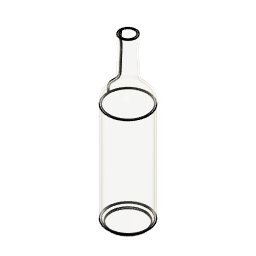
Glass_bottle_ (Autodesk Fusion 360 design; units mm, degrees)
Autodesk Fusion 360 part; units mm, degrees
sketch "Sketch1" plane through (0, 0, 0) normal (0, 1, 0) x (1, 0, 0)
  line L0 (0, 0) -> (0, -240)
  line L1 (0, 0) -> (-29.692, 0)
  line L2 (-29.692, 0) -> (-29.692, -150)
  spline S0 degree 5 poles (-29.692, -150) (-29.8152, -150.759) (-30.0072, -152.2507) (-30.1322, -154.409) (-29.9719, -157.1282) (-29.2328, -160.2645) (-27.979, -163.1461) (-26.2639, -165.7913) (-24.179, -168.2327) (-21.8712, -170.5218) (-19.5246, -172.7277) (-17.3289, -174.9305) (-15.4503, -177.2171) (-14.0044, -179.6762) (-13.0199, -182.3939) (-12.439, -185.4454) (-12.1537, -188.882) (-12.0325, -192.7196) (-11.9509, -196.9254) (-11.8186, -201.4068) (-11.6132, -205.9935) (-11.3668, -210.4677) (-11.141, -214.6054) (-11.0072, -218.2126) (-11.0231, -221.1668) (-11.2145, -223.4494) (-11.5459, -225.2013) (-11.9243, -226.7037) (-12.2401, -228.2746) (-12.4028, -230.1713) (-12.3627, -232.5371) (-12.1483, -234.8625) (-11.8818, -236.8594) (-11.6572, -238.3028) (-11.5332, -239.0525) knots 0 0 0 0 0 0 0.033333 0.066667 0.1 0.133333 0.166667 0.2 0.233333 0.266667 0.3 0.333333 0.366667 0.4 0.433333 0.466667 0.5 0.533333 0.566667 0.6 0.633333 0.666667 0.7 0.733333 0.766667 0.8 0.833333 0.866667 0.9 0.933333 0.966667 1 1 1 1 1 1
  line L3 (0, -240) -> (-11.5332, -239.0525)
  line L4 (-11.5332, -239.0525) -> (0, -240)
  point P0 (-25.5317, -166.5673)
  point P1 (-14.7931, -178.4564)
  point P2 (-11.9168, -197.8242)
  point P3 (-11.1497, -222.3694)
  point P4 (-12.1085, -227.7387)
  constraint coincident L0.start L1.start
  constraint vertical L0
  constraint perpendicular L0 L1
  constraint perpendicular L1 L2
revolve "Revolve1" add sketch "Sketch1" angle 360 about axis through (0, 0, 0) along (0, 0, 1)
fillet "Fillet1" radius 5 1 edges at (-27.6826, 10.7371, 0)
shell "Shell1" thickness 2 removed faces 1 at (-8.7096, 2.1467, 239.2631)
